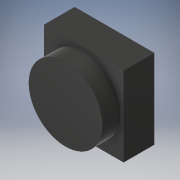
# Autodesk Inventor part: CameraLens
Saved by Autodesk Inventor 2018 (Build 220112000, 112)
## iProperties
Created: 2018-01-13
Part Number: CameraLens
Material: ABS Plastic
Document SubType Name: Modeling
Designer: Kyle-HP
Density: 1.06 g/cm^3
Appearance: Smooth - Black
Author: Kyle-HP
Autodesk Inventor part; units mm, degrees
ref_plane "YZ Plane" through (0, 0, 0) normal (1, 0, 0) x (0, 1, 0)
ref_plane "XZ Plane" through (0, 0, 0) normal (0, 1, 0) x (-1, 0, 0)
ref_plane "XY Plane" through (0, 0, 0) normal (0, 0, 1) x (1, 0, 0)
sketch "Sketch1" plane through (0, 0, 0) normal (0, 0, 1) x (1, 0, 0)
  line L0 (0, 0) -> (8.255, 0)
  line L1 (8.255, 0) -> (8.255, -8.255)
  line L2 (8.255, -8.255) -> (0, -8.255)
  line L3 (0, -8.255) -> (0, 0)
  dimension "d0" = 8.255
  dimension "d1" = 8.255
  constraints: 8 end point, 2 parallel, 1 horizontal, 1 perpendicular
  measures "d0" distance of L0.start L0.end
  measures "d1" distance of L0.end L1.end
extrude "Extrusion1" add sketch "Sketch1" along normal blind 3.175
sketch "Sketch2" plane through (0, 0, 3.175) normal (0, 0, 1) x (1, 0, 0)
  circle A0 centre (4.1275, -4.1275) radius 3.81
  line L0 (0, 0) -> (0, -8.255) projected
  line L1 (8.255, 0) -> (0, 0) projected
  dimension "d4" = 7.62
  dimension "d5" = 4.1275
  dimension "d6" = 4.1275
  constraints: 1 centre point
  measures "d4" diameter of A0
  measures "d5" distance from line of L0 A0.centre
  measures "d6" distance from line of L1 A0.centre
extrude "Extrusion2" add sketch "Sketch2" along normal blind 1.905
body "Solid1"
